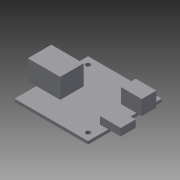
# Autodesk Inventor part: PCB-Model
Saved by Autodesk Inventor 2013 (Build 170138000, 138)
## iProperties
Created: 2013-01-07
Part Number: PCB-Model
Material: Generic
Document SubType Name: Modeling
Designer: md
Density: 1 g/cm^3
Author: md
Autodesk Inventor part; units mm, degrees
ref_plane "YZ Plane" through (0, 0, 0) normal (1, 0, 0) x (0, 1, 0)
ref_plane "XZ Plane" through (0, 0, 0) normal (0, 1, 0) x (-1, 0, 0)
ref_plane "XY Plane" through (0, 0, 0) normal (0, 0, 1) x (1, 0, 0)
sketch "Platine" plane through (0, 0, 0) normal (0, 0, 1) x (1, 0, 0)
  line L0 (-25, -25) -> (25, -25)
  line L1 (25, -25) -> (25, 25)
  line L2 (25, 25) -> (-25, 25)
  line L3 (-25, 25) -> (-25, -25)
  line L4 (-25, -25) -> (25, 25)
  line L5 (25, -25) -> (-25, 25)
  line L6 (-30.8, -10.2) -> (-8.8, -10.2)
  line L7 (-8.8, -10.2) -> (-8.8, 5.8)
  line L8 (-8.8, 5.8) -> (-30.8, 5.8)
  line L9 (-30.8, 5.8) -> (-30.8, -10.2)
  line L10 (33.4, -11.2) -> (19.4, -11.2)
  line L11 (19.4, -11.2) -> (19.4, -1.04)
  line L12 (19.4, -1.04) -> (33.4, -1.04)
  line L13 (33.4, -1.04) -> (33.4, -11.2)
  line L14 (14.5, 8) -> (28.5, 8)
  line L15 (28.5, 8) -> (28.5, 18)
  line L16 (28.5, 18) -> (14.5, 18)
  line L17 (14.5, 18) -> (14.5, 8)
  circle A0 centre (-20, 20) radius 1.5
  circle A1 centre (20, -20) radius 1.5
  point P0 (0, 0)
  point P1 (0, 0)
  dimension "d0" = 50
  dimension "d1" = 50
  dimension "d2" = 22
  dimension "d3" = 16
  dimension "d4" = 14.8
  dimension "d5" = 5.8
  dimension "d6" = 14
  dimension "d7" = 10.16
  dimension "d8" = 13.8
  dimension "d9" = 44.4
  dimension "d10" = 10
  dimension "d11" = 14
  dimension "d12" = 33
  dimension "d13" = 10.5
  dimension "d14" = 3
  dimension "d15" = 5
  dimension "d16" = 5
  dimension "d17" = 5
  dimension "d18" = 5
  dimension "d19" = 18
  dimension "d20" = 33.4
  constraints: 36 end point, 8 parallel, 4 horizontal, 4 perpendicular, 2 centre point, 2 midpoint, 1 equal radius
  measures "d0" distance between parallel lines of L0 L2
  measures "d1" distance between parallel lines of L1 L3
  measures "d2" distance between parallel lines of L7 L9
  measures "d3" distance of L8.end L6.start
  measures "d4" distance between parallel lines of L6 L0
  measures "d5" distance between parallel lines of L9 L3
  measures "d6" distance between parallel lines of L13 L11
  measures "d7" distance between parallel lines of L10 L12
  measures "d8" distance between parallel lines of L0 L10
  measures "d9" distance between parallel lines of L3 L11
  measures "d10" distance between parallel lines of L14 L16
  measures "d11" distance between parallel lines of L15 L17
  measures "d12" distance between parallel lines of L0 L14
  measures "d13" distance between parallel lines of L1 L17
  measures "d14" diameter of A0
  measures "d15" distance from line of A0.centre L3
  measures "d16" distance from line of A0.centre L2
  measures "d17" distance from line of A1.centre L1
  measures "d18" distance from line of A1.centre L0
  measures "d19" distance from line of point (0, 0) L16
  measures "d20" distance from line of point (0, 0) L13
extrude "Platinengeometrie" add sketch "Platine" against normal blind 2 contours L4 L6 L7 L5 A1 L0 | L3 L6 L4 | L5 A1 L4 L17 L14 L1 L12 L11 L10 | L3 L8 L7 L4 L6 | L4 L7 L6 | L10 L11 L12 L1 | A1 L5 | L5 A1 | L3 L5 A0 L4 L7 L8 | L2 L4 L16 L17 L5 A0 | L14 L17 L4 L16 L1 | L1 L16 L4 | A0 L5 | L5 A0 | L17 L16 L4
sketch "Platine2" plane through (0, 0, 0) normal (0, 0, 1) x (1, 0, 0)
  line L0 (-25, -25) -> (25, -25)
  line L1 (25, -25) -> (25, 25)
  line L2 (25, 25) -> (-25, 25)
  line L3 (-25, 25) -> (-25, -25)
  line L4 (-25, -25) -> (25, 25)
  line L5 (25, -25) -> (-25, 25)
  line L6 (-30.8, -10.2) -> (-8.8, -10.2)
  line L7 (-8.8, -10.2) -> (-8.8, 5.8)
  line L8 (-8.8, 5.8) -> (-30.8, 5.8)
  line L9 (-30.8, 5.8) -> (-30.8, -10.2)
  line L10 (33.4, -11.2) -> (19.4, -11.2)
  line L11 (19.4, -11.2) -> (19.4, -1.04)
  line L12 (19.4, -1.04) -> (33.4, -1.04)
  line L13 (33.4, -1.04) -> (33.4, -11.2)
  line L14 (14.5, 8) -> (28.5, 8)
  line L15 (28.5, 8) -> (28.5, 18)
  line L16 (28.5, 18) -> (14.5, 18)
  line L17 (14.5, 18) -> (14.5, 8)
  circle A0 centre (-20, 20) radius 1.5
  circle A1 centre (20, -20) radius 1.5
  point P0 (0, 0)
  point P1 (0, 0)
  point P2 (0, 0)
  dimension "d23" = 50
  dimension "d24" = 50
  dimension "d25" = 22
  dimension "d26" = 16
  dimension "d27" = 14.8
  dimension "d28" = 5.8
  dimension "d29" = 14
  dimension "d30" = 10.16
  dimension "d31" = 13.8
  dimension "d32" = 44.4
  dimension "d33" = 10
  dimension "d34" = 14
  dimension "d35" = 33
  dimension "d36" = 10.5
  dimension "d37" = 3
  dimension "d38" = 5
  dimension "d39" = 5
  dimension "d40" = 5
  dimension "d41" = 5
  dimension "d42" = 18
  dimension "d43" = 33.4
  constraints: 36 end point, 8 parallel, 4 horizontal, 4 perpendicular, 2 centre point, 2 midpoint, 1 equal radius
  measures "d23" distance between parallel lines of L0 L2
  measures "d24" distance between parallel lines of L1 L3
  measures "d25" distance between parallel lines of L7 L9
  measures "d26" distance of L8.end L6.start
  measures "d27" distance between parallel lines of L6 L0
  measures "d28" distance between parallel lines of L9 L3
  measures "d29" distance between parallel lines of L13 L11
  measures "d30" distance between parallel lines of L10 L12
  measures "d31" distance between parallel lines of L0 L10
  measures "d32" distance between parallel lines of L3 L11
  measures "d33" distance between parallel lines of L14 L16
  measures "d34" distance between parallel lines of L15 L17
  measures "d35" distance between parallel lines of L0 L14
  measures "d36" distance between parallel lines of L1 L17
  measures "d37" diameter of A0
  measures "d38" distance from line of A0.centre L3
  measures "d39" distance from line of A0.centre L2
  measures "d40" distance from line of A1.centre L1
  measures "d41" distance from line of A1.centre L0
  measures "d42" distance from line of point (0, 0) L16
  measures "d43" distance from line of point (0, 0) L13
extrude "MEBP 8-8G" add sketch "Platine2" along normal blind 13.5 contours L6 L9 L8 L3 | L3 L8 L7 L4 L6 | L4 L7 L6
sketch "Platine3" plane through (0, 0, 0) normal (0, 0, 1) x (1, 0, 0)
  line L0 (-25, -25) -> (25, -25)
  line L1 (25, -25) -> (25, 25)
  line L2 (25, 25) -> (-25, 25)
  line L3 (-25, 25) -> (-25, -25)
  line L4 (-25, -25) -> (25, 25)
  line L5 (25, -25) -> (-25, 25)
  line L6 (-30.8, -10.2) -> (-8.8, -10.2)
  line L7 (-8.8, -10.2) -> (-8.8, 5.8)
  line L8 (-8.8, 5.8) -> (-30.8, 5.8)
  line L9 (-30.8, 5.8) -> (-30.8, -10.2)
  line L10 (33.4, -11.2) -> (19.4, -11.2)
  line L11 (19.4, -11.2) -> (19.4, -1.04)
  line L12 (19.4, -1.04) -> (33.4, -1.04)
  line L13 (33.4, -1.04) -> (33.4, -11.2)
  line L14 (14.5, 8) -> (28.5, 8)
  line L15 (28.5, 8) -> (28.5, 18)
  line L16 (28.5, 18) -> (14.5, 18)
  line L17 (14.5, 18) -> (14.5, 8)
  circle A0 centre (-20, 20) radius 1.5
  circle A1 centre (20, -20) radius 1.5
  point P0 (0, 0)
  point P1 (0, 0)
  point P2 (0, 0)
  dimension "d46" = 50
  dimension "d47" = 50
  dimension "d48" = 22
  dimension "d49" = 16
  dimension "d50" = 14.8
  dimension "d51" = 5.8
  dimension "d52" = 14
  dimension "d53" = 10.16
  dimension "d54" = 13.8
  dimension "d55" = 44.4
  dimension "d56" = 10
  dimension "d57" = 14
  dimension "d58" = 33
  dimension "d59" = 10.5
  dimension "d60" = 3
  dimension "d61" = 5
  dimension "d62" = 5
  dimension "d63" = 5
  dimension "d64" = 5
  dimension "d65" = 18
  dimension "d66" = 33.4
  constraints: 36 end point, 8 parallel, 4 horizontal, 4 perpendicular, 2 centre point, 2 midpoint, 1 equal radius
  measures "d46" distance between parallel lines of L0 L2
  measures "d47" distance between parallel lines of L1 L3
  measures "d48" distance between parallel lines of L7 L9
  measures "d49" distance of L8.end L6.start
  measures "d50" distance between parallel lines of L6 L0
  measures "d51" distance between parallel lines of L9 L3
  measures "d52" distance between parallel lines of L13 L11
  measures "d53" distance between parallel lines of L10 L12
  measures "d54" distance between parallel lines of L0 L10
  measures "d55" distance between parallel lines of L3 L11
  measures "d56" distance between parallel lines of L14 L16
  measures "d57" distance between parallel lines of L15 L17
  measures "d58" distance between parallel lines of L0 L14
  measures "d59" distance between parallel lines of L1 L17
  measures "d60" diameter of A0
  measures "d61" distance from line of A0.centre L3
  measures "d62" distance from line of A0.centre L2
  measures "d63" distance from line of A1.centre L1
  measures "d64" distance from line of A1.centre L0
  measures "d65" distance from line of point (0, 0) L16
  measures "d66" distance from line of point (0, 0) L13
extrude "PSS 254/4W" add sketch "Platine3" along normal blind 5 contours L10 L11 L12 L1 | L1 L12 L13 L10
sketch "Sketch4" plane through (0, 0, 0) normal (0, 0, 1) x (1, 0, 0)
  line L0 (-25, -25) -> (25, -25)
  line L1 (25, -25) -> (25, 25)
  line L2 (25, 25) -> (-25, 25)
  line L3 (-25, 25) -> (-25, -25)
  line L4 (-25, -25) -> (25, 25)
  line L5 (25, -25) -> (-25, 25)
  line L6 (-30.8, -10.2) -> (-8.8, -10.2)
  line L7 (-8.8, -10.2) -> (-8.8, 5.8)
  line L8 (-8.8, 5.8) -> (-30.8, 5.8)
  line L9 (-30.8, 5.8) -> (-30.8, -10.2)
  line L10 (33.4, -11.2) -> (19.4, -11.2)
  line L11 (19.4, -11.2) -> (19.4, -1.04)
  line L12 (19.4, -1.04) -> (33.4, -1.04)
  line L13 (33.4, -1.04) -> (33.4, -11.2)
  line L14 (14.5, 8) -> (28.5, 8)
  line L15 (28.5, 8) -> (28.5, 18)
  line L16 (28.5, 18) -> (14.5, 18)
  line L17 (14.5, 18) -> (14.5, 8)
  circle A0 centre (-20, 20) radius 1.5
  circle A1 centre (20, -20) radius 1.5
  point P0 (0, 0)
  point P1 (0, 0)
  point P2 (0, 0)
  dimension "d69" = 50
  dimension "d70" = 50
  dimension "d71" = 22
  dimension "d72" = 16
  dimension "d73" = 14.8
  dimension "d74" = 5.8
  dimension "d75" = 14
  dimension "d76" = 10.16
  dimension "d77" = 13.8
  dimension "d78" = 44.4
  dimension "d79" = 10
  dimension "d80" = 14
  dimension "d81" = 33
  dimension "d82" = 10.5
  dimension "d83" = 3
  dimension "d84" = 5
  dimension "d85" = 5
  dimension "d86" = 5
  dimension "d87" = 5
  dimension "d88" = 18
  dimension "d89" = 33.4
  constraints: 36 end point, 8 parallel, 4 horizontal, 4 perpendicular, 2 centre point, 2 midpoint, 1 equal radius
  measures "d69" distance between parallel lines of L0 L2
  measures "d70" distance between parallel lines of L1 L3
  measures "d71" distance between parallel lines of L7 L9
  measures "d72" distance of L8.end L6.start
  measures "d73" distance between parallel lines of L6 L0
  measures "d74" distance between parallel lines of L9 L3
  measures "d75" distance between parallel lines of L13 L11
  measures "d76" distance between parallel lines of L10 L12
  measures "d77" distance between parallel lines of L0 L10
  measures "d78" distance between parallel lines of L3 L11
  measures "d79" distance between parallel lines of L14 L16
  measures "d80" distance between parallel lines of L15 L17
  measures "d81" distance between parallel lines of L0 L14
  measures "d82" distance between parallel lines of L1 L17
  measures "d83" diameter of A0
  measures "d84" distance from line of A0.centre L3
  measures "d85" distance from line of A0.centre L2
  measures "d86" distance from line of A1.centre L1
  measures "d87" distance from line of A1.centre L0
  measures "d88" distance from line of point (0, 0) L16
  measures "d89" distance from line of point (0, 0) L13
extrude "HEBG9 25" add sketch "Sketch4" along normal blind 10 contours L14 L17 L4 L16 L1 | L1 L16 L15 L14 | L17 L16 L4
sketch "Sketch5" plane through (0, 0, 0) normal (0, 0, 1) x (1, 0, 0)
  line L0 (-25, -25) -> (25, -25)
  line L1 (25, -25) -> (25, 25)
  line L2 (25, 25) -> (-25, 25)
  line L3 (-25, 25) -> (-25, -25)
  line L4 (-25, -25) -> (25, 25)
  line L5 (25, -25) -> (-25, 25)
  line L6 (-30.8, -10.2) -> (-8.8, -10.2)
  line L7 (-8.8, -10.2) -> (-8.8, 5.8)
  line L8 (-8.8, 5.8) -> (-30.8, 5.8)
  line L9 (-30.8, 5.8) -> (-30.8, -10.2)
  line L10 (33.4, -11.2) -> (19.4, -11.2)
  line L11 (19.4, -11.2) -> (19.4, -1.04)
  line L12 (19.4, -1.04) -> (33.4, -1.04)
  line L13 (33.4, -1.04) -> (33.4, -11.2)
  line L14 (14.5, 8) -> (28.5, 8)
  line L15 (28.5, 8) -> (28.5, 18)
  line L16 (28.5, 18) -> (14.5, 18)
  line L17 (14.5, 18) -> (14.5, 8)
  circle A0 centre (-20, 20) radius 1.5
  circle A1 centre (20, -20) radius 1.5
  point P0 (0, 0)
  point P1 (0, 0)
  point P2 (0, 0)
  dimension "d92" = 50
  dimension "d93" = 50
  dimension "d94" = 22
  dimension "d95" = 16
  dimension "d96" = 14.8
  dimension "d97" = 5.8
  dimension "d98" = 14
  dimension "d99" = 10.16
  dimension "d100" = 13.8
  dimension "d101" = 44.4
  dimension "d102" = 10
  dimension "d103" = 14
  dimension "d104" = 33
  dimension "d105" = 10.5
  dimension "d106" = 3
  dimension "d107" = 5
  dimension "d108" = 5
  dimension "d109" = 5
  dimension "d110" = 5
  dimension "d111" = 18
  dimension "d112" = 33.4
  constraints: 36 end point, 8 parallel, 4 horizontal, 4 perpendicular, 2 centre point, 2 midpoint, 1 equal radius
  measures "d92" distance between parallel lines of L0 L2
  measures "d93" distance between parallel lines of L1 L3
  measures "d94" distance between parallel lines of L7 L9
  measures "d95" distance of L8.end L6.start
  measures "d96" distance between parallel lines of L6 L0
  measures "d97" distance between parallel lines of L9 L3
  measures "d98" distance between parallel lines of L13 L11
  measures "d99" distance between parallel lines of L10 L12
  measures "d100" distance between parallel lines of L0 L10
  measures "d101" distance between parallel lines of L3 L11
  measures "d102" distance between parallel lines of L14 L16
  measures "d103" distance between parallel lines of L15 L17
  measures "d104" distance between parallel lines of L0 L14
  measures "d105" distance between parallel lines of L1 L17
  measures "d106" diameter of A0
  measures "d107" distance from line of A0.centre L3
  measures "d108" distance from line of A0.centre L2
  measures "d109" distance from line of A1.centre L1
  measures "d110" distance from line of A1.centre L0
  measures "d111" distance from line of point (0, 0) L16
  measures "d112" distance from line of point (0, 0) L13
hole "Hole1" at (-20, 20, 0) at (20, -20, 0) direction (0, 0, -1) diameter 3.1 end through all
